Autodesk Fusion 360 part; units mm, degrees
(part 2 of 2)
sketch "Sketch2 (2)" plane through (0, 0, 0) normal (0, 0, 1) x (1, 0, 0) in component "Spur Gear (8 teeth)"
  spline S0 degree 5 poles (4.6675, -1.001) (4.6721, -1.0019) (4.6813, -1.0037) (4.6952, -1.0059) (4.7138, -1.0078) (4.7373, -1.0088) (4.7609, -1.0089) (4.7846, -1.0084) (4.8084, -1.0076) (4.8323, -1.0065) (4.8562, -1.0051) (4.8801, -1.0035) (4.9041, -1.0014) (4.9282, -0.9988) (4.9523, -0.9957) (4.9764, -0.9922) (5.0006, -0.9883) (5.0248, -0.9841) (5.049, -0.9795) (5.0733, -0.9747) (5.0975, -0.9696) (5.1218, -0.9642) (5.1461, -0.9584) (5.1705, -0.9524) (5.1948, -0.946) (5.2191, -0.9393) (5.2435, -0.9324) (5.2679, -0.9251) (5.2922, -0.9176) (5.3166, -0.9098) (5.3409, -0.9017) (5.3653, -0.8934) (5.3896, -0.8848) (5.414, -0.8759) (5.4383, -0.8668) (5.4626, -0.8574) (5.4869, -0.8477) (5.5112, -0.8378) (5.5355, -0.8277) (5.5598, -0.8173) (5.584, -0.8066) (5.6082, -0.7957) (5.6324, -0.7845) (5.6566, -0.7731) (5.6808, -0.7615) (5.7049, -0.7496) (5.729, -0.7375) (5.7531, -0.7252) (5.7771, -0.7126) (5.8011, -0.6997) (5.825, -0.6867) (5.849, -0.6734) (5.8729, -0.6599) (5.8967, -0.6462) (5.9205, -0.6322) (5.9443, -0.618) (5.968, -0.6036) (5.9917, -0.589) (6.0153, -0.5741) (6.0389, -0.559) (6.0625, -0.5438) (6.086, -0.5282) (6.1094, -0.5125) (6.1328, -0.4966) (6.1561, -0.4804) (6.1794, -0.464) (6.2026, -0.4475) (6.2258, -0.4307) (6.2489, -0.4137) (6.2719, -0.3965) (6.2949, -0.379) (6.3133, -0.3649) (6.327, -0.3543) (6.3361, -0.3471) (6.3407, -0.3435) knots 0 0 0 0 0 0 0.01428571 0.02857143 0.04285714 0.05714286 0.07142857 0.08571429 0.1 0.11428571 0.12857143 0.14285714 0.15714286 0.17142857 0.18571429 0.2 0.21428571 0.22857143 0.24285714 0.25714286 0.27142857 0.28571429 0.3 0.31428571 0.32857143 0.34285714 0.35714286 0.37142857 0.38571429 0.4 0.41428571 0.42857143 0.44285714 0.45714286 0.47142857 0.48571429 0.5 0.51428571 0.52857143 0.54285714 0.55714286 0.57142857 0.58571429 0.6 0.61428571 0.62857143 0.64285714 0.65714286 0.67142857 0.68571429 0.7 0.71428571 0.72857143 0.74285714 0.75714286 0.77142857 0.78571429 0.8 0.81428571 0.82857143 0.84285714 0.85714286 0.87142857 0.88571429 0.9 0.91428571 0.92857143 0.94285714 0.95714286 0.97142857 0.98571429 1 1 1 1 1 1
  spline S1 degree 5 poles (4.6675, 1.001) (4.6721, 1.0019) (4.6813, 1.0037) (4.6952, 1.0059) (4.7138, 1.0078) (4.7373, 1.0088) (4.7609, 1.0089) (4.7846, 1.0084) (4.8084, 1.0076) (4.8323, 1.0065) (4.8562, 1.0051) (4.8801, 1.0035) (4.9041, 1.0014) (4.9282, 0.9988) (4.9523, 0.9957) (4.9764, 0.9922) (5.0006, 0.9883) (5.0248, 0.9841) (5.049, 0.9795) (5.0733, 0.9747) (5.0975, 0.9696) (5.1218, 0.9642) (5.1461, 0.9584) (5.1705, 0.9524) (5.1948, 0.946) (5.2191, 0.9393) (5.2435, 0.9324) (5.2679, 0.9251) (5.2922, 0.9176) (5.3166, 0.9098) (5.3409, 0.9017) (5.3653, 0.8934) (5.3896, 0.8848) (5.414, 0.8759) (5.4383, 0.8668) (5.4626, 0.8574) (5.4869, 0.8477) (5.5112, 0.8378) (5.5355, 0.8277) (5.5598, 0.8173) (5.584, 0.8066) (5.6082, 0.7957) (5.6324, 0.7845) (5.6566, 0.7731) (5.6808, 0.7615) (5.7049, 0.7496) (5.729, 0.7375) (5.7531, 0.7252) (5.7771, 0.7126) (5.8011, 0.6997) (5.825, 0.6867) (5.849, 0.6734) (5.8729, 0.6599) (5.8967, 0.6462) (5.9205, 0.6322) (5.9443, 0.618) (5.968, 0.6036) (5.9917, 0.589) (6.0153, 0.5741) (6.0389, 0.559) (6.0625, 0.5438) (6.086, 0.5282) (6.1094, 0.5125) (6.1328, 0.4966) (6.1561, 0.4804) (6.1794, 0.464) (6.2026, 0.4475) (6.2258, 0.4307) (6.2489, 0.4137) (6.2719, 0.3965) (6.2949, 0.379) (6.3133, 0.3649) (6.327, 0.3543) (6.3361, 0.3471) (6.3407, 0.3435) knots 0 0 0 0 0 0 0.01428571 0.02857143 0.04285714 0.05714286 0.07142857 0.08571429 0.1 0.11428571 0.12857143 0.14285714 0.15714286 0.17142857 0.18571429 0.2 0.21428571 0.22857143 0.24285714 0.25714286 0.27142857 0.28571429 0.3 0.31428571 0.32857143 0.34285714 0.35714286 0.37142857 0.38571429 0.4 0.41428571 0.42857143 0.44285714 0.45714286 0.47142857 0.48571429 0.5 0.51428571 0.52857143 0.54285714 0.55714286 0.57142857 0.58571429 0.6 0.61428571 0.62857143 0.64285714 0.65714286 0.67142857 0.68571429 0.7 0.71428571 0.72857143 0.74285714 0.75714286 0.77142857 0.78571429 0.8 0.81428571 0.82857143 0.84285714 0.85714286 0.87142857 0.88571429 0.9 0.91428571 0.92857143 0.94285714 0.95714286 0.97142857 0.98571429 1 1 1 1 1 1
  arc A0 (6.3407, -0.3435) -> (6.3407, 0.3435) centre (0, 0) ccw
  line L0 (3.4175, -0.735) -> (4.6675, -1.001)
  line L1 (3.4175, 0.735) -> (4.6675, 1.001)
  line L2 (3.4175, -0.735) -> (3.4175, 0.735)
  point P0 (4.781, -1.0084)
  point P1 (4.8974, -1.0019)
  point P2 (5.0155, -0.9856)
  point P3 (5.1349, -0.961)
  point P4 (5.2552, -0.9289)
  point P5 (5.3761, -0.8895)
  point P6 (5.4975, -0.8434)
  point P7 (5.6191, -0.7907)
  point P8 (5.7406, -0.7315)
  point P9 (5.8619, -0.6661)
  point P10 (5.9827, -0.5945)
  point P11 (6.103, -0.5168)
  point P12 (6.2223, -0.4331)
  point P13 (4.781, 1.0084)
  point P14 (4.8974, 1.0019)
  point P15 (5.0155, 0.9856)
  point P16 (5.1349, 0.961)
  point P17 (5.2552, 0.9289)
  point P18 (5.3761, 0.8895)
  point P19 (5.4975, 0.8434)
  point P20 (5.6191, 0.7907)
  point P21 (5.7406, 0.7315)
  point P22 (5.8619, 0.6661)
  point P23 (5.9827, 0.5945)
  point P24 (6.103, 0.5168)
  point P25 (6.2223, 0.4331)
extrude "Extrude2" add sketch "Sketch2 (2)" along normal blind 7.62 in component "Spur Gear (8 teeth)"
fillet "Fillet1" radius 0.254 2 edges at (3.4268, -0.737, 3.81) (3.4268, 0.737, 3.81) in component "Spur Gear (8 teeth)"
pattern_circular "C-Pattern1" count 8 over 360 about axis through (0, 0, 0) along (0, 0, 1) of "Extrude2", "Fillet1" in component "Spur Gear (8 teeth)"
sketch "Sketch3" plane through (0, 0, 0) normal (0, 0, 1) x (1, 0, 0) in component "Spur Gear (8 teeth)"
  circle A0 centre (0, 0) radius 5.08 construction
sketch "Sketch3 (2)" plane through (0, 0, 0) normal (0, 0, -1) x (-1, 0, 0)
  circle A0 centre (0, 0) radius 3.175
  arc A1 (-0.7879, -3.6664) -> (-0.9664, -3.3694) centre (-1.0364, -3.6135) ccw
  line L0 (-0.7879, -3.6664) -> (-1.001, -4.6675)
  spline S0 degree 5 poles (-1.001, -4.6675) (-1.0019, -4.6721) (-1.0037, -4.6813) (-1.0059, -4.6952) (-1.0078, -4.7138) (-1.0088, -4.7373) (-1.0089, -4.7609) (-1.0084, -4.7846) (-1.0076, -4.8084) (-1.0065, -4.8323) (-1.0051, -4.8562) (-1.0035, -4.8801) (-1.0014, -4.9041) (-0.9988, -4.9282) (-0.9957, -4.9523) (-0.9922, -4.9764) (-0.9883, -5.0006) (-0.9841, -5.0248) (-0.9795, -5.049) (-0.9747, -5.0733) (-0.9696, -5.0975) (-0.9642, -5.1218) (-0.9584, -5.1461) (-0.9524, -5.1705) (-0.946, -5.1948) (-0.9393, -5.2191) (-0.9324, -5.2435) (-0.9251, -5.2679) (-0.9176, -5.2922) (-0.9098, -5.3166) (-0.9017, -5.3409) (-0.8934, -5.3653) (-0.8848, -5.3896) (-0.8759, -5.414) (-0.8668, -5.4383) (-0.8574, -5.4626) (-0.8477, -5.4869) (-0.8378, -5.5112) (-0.8277, -5.5355) (-0.8173, -5.5598) (-0.8066, -5.584) (-0.7957, -5.6082) (-0.7845, -5.6324) (-0.7731, -5.6566) (-0.7615, -5.6808) (-0.7496, -5.7049) (-0.7375, -5.729) (-0.7252, -5.7531) (-0.7126, -5.7771) (-0.6997, -5.8011) (-0.6867, -5.825) (-0.6734, -5.849) (-0.6599, -5.8729) (-0.6462, -5.8967) (-0.6322, -5.9205) (-0.618, -5.9443) (-0.6036, -5.968) (-0.589, -5.9917) (-0.5741, -6.0153) (-0.559, -6.0389) (-0.5438, -6.0625) (-0.5282, -6.086) (-0.5125, -6.1094) (-0.4966, -6.1328) (-0.4804, -6.1561) (-0.464, -6.1794) (-0.4475, -6.2026) (-0.4307, -6.2258) (-0.4137, -6.2489) (-0.3965, -6.2719) (-0.379, -6.2949) (-0.3649, -6.3133) (-0.3543, -6.327) (-0.3471, -6.3361) (-0.3435, -6.3407) knots 0 0 0 0 0 0 0.01428571 0.02857143 0.04285714 0.05714286 0.07142857 0.08571429 0.1 0.11428571 0.12857143 0.14285714 0.15714286 0.17142857 0.18571429 0.2 0.21428571 0.22857143 0.24285714 0.25714286 0.27142857 0.28571429 0.3 0.31428571 0.32857143 0.34285714 0.35714286 0.37142857 0.38571429 0.4 0.41428571 0.42857143 0.44285714 0.45714286 0.47142857 0.48571429 0.5 0.51428571 0.52857143 0.54285714 0.55714286 0.57142857 0.58571429 0.6 0.61428571 0.62857143 0.64285714 0.65714286 0.67142857 0.68571429 0.7 0.71428571 0.72857143 0.74285714 0.75714286 0.77142857 0.78571429 0.8 0.81428571 0.82857143 0.84285714 0.85714286 0.87142857 0.88571429 0.9 0.91428571 0.92857143 0.94285714 0.95714286 0.97142857 0.98571429 1 1 1 1 1 1
  arc A2 (-0.3435, -6.3407) -> (0.3435, -6.3407) centre (0, 0) ccw
  spline S1 degree 5 poles (1.001, -4.6675) (1.0019, -4.6721) (1.0037, -4.6813) (1.0059, -4.6952) (1.0078, -4.7138) (1.0088, -4.7373) (1.0089, -4.7609) (1.0084, -4.7846) (1.0076, -4.8084) (1.0065, -4.8323) (1.0051, -4.8562) (1.0035, -4.8801) (1.0014, -4.9041) (0.9988, -4.9282) (0.9957, -4.9523) (0.9922, -4.9764) (0.9883, -5.0006) (0.9841, -5.0248) (0.9795, -5.049) (0.9747, -5.0733) (0.9696, -5.0975) (0.9642, -5.1218) (0.9584, -5.1461) (0.9524, -5.1705) (0.946, -5.1948) (0.9393, -5.2191) (0.9324, -5.2435) (0.9251, -5.2679) (0.9176, -5.2922) (0.9098, -5.3166) (0.9017, -5.3409) (0.8934, -5.3653) (0.8848, -5.3896) (0.8759, -5.414) (0.8668, -5.4383) (0.8574, -5.4626) (0.8477, -5.4869) (0.8378, -5.5112) (0.8277, -5.5355) (0.8173, -5.5598) (0.8066, -5.584) (0.7957, -5.6082) (0.7845, -5.6324) (0.7731, -5.6566) (0.7615, -5.6808) (0.7496, -5.7049) (0.7375, -5.729) (0.7252, -5.7531) (0.7126, -5.7771) (0.6997, -5.8011) (0.6867, -5.825) (0.6734, -5.849) (0.6599, -5.8729) (0.6462, -5.8967) (0.6322, -5.9205) (0.618, -5.9443) (0.6036, -5.968) (0.589, -5.9917) (0.5741, -6.0153) (0.559, -6.0389) (0.5438, -6.0625) (0.5282, -6.086) (0.5125, -6.1094) (0.4966, -6.1328) (0.4804, -6.1561) (0.464, -6.1794) (0.4475, -6.2026) (0.4307, -6.2258) (0.4137, -6.2489) (0.3965, -6.2719) (0.379, -6.2949) (0.3649, -6.3133) (0.3543, -6.327) (0.3471, -6.3361) (0.3435, -6.3407) knots 0 0 0 0 0 0 0.01428571 0.02857143 0.04285714 0.05714286 0.07142857 0.08571429 0.1 0.11428571 0.12857143 0.14285714 0.15714286 0.17142857 0.18571429 0.2 0.21428571 0.22857143 0.24285714 0.25714286 0.27142857 0.28571429 0.3 0.31428571 0.32857143 0.34285714 0.35714286 0.37142857 0.38571429 0.4 0.41428571 0.42857143 0.44285714 0.45714286 0.47142857 0.48571429 0.5 0.51428571 0.52857143 0.54285714 0.55714286 0.57142857 0.58571429 0.6 0.61428571 0.62857143 0.64285714 0.65714286 0.67142857 0.68571429 0.7 0.71428571 0.72857143 0.74285714 0.75714286 0.77142857 0.78571429 0.8 0.81428571 0.82857143 0.84285714 0.85714286 0.87142857 0.88571429 0.9 0.91428571 0.92857143 0.94285714 0.95714286 0.97142857 0.98571429 1 1 1 1 1 1
  line L1 (1.001, -4.6675) -> (0.7879, -3.6664)
  arc A3 (0.9664, -3.3694) -> (0.7879, -3.6664) centre (1.0364, -3.6135) ccw
  arc A4 (0.9664, -3.3694) -> (1.6992, -3.0658) centre (0, 0) ccw
  arc A5 (2.0354, -3.1497) -> (1.6992, -3.0658) centre (1.8223, -3.288) ccw
  line L2 (2.0354, -3.1497) -> (2.5926, -4.0082)
  spline S2 degree 5 poles (2.5926, -4.0082) (2.5952, -4.0122) (2.6004, -4.0199) (2.6087, -4.0313) (2.6205, -4.0458) (2.6364, -4.0631) (2.6531, -4.0799) (2.6702, -4.0963) (2.6876, -4.1125) (2.7053, -4.1286) (2.7231, -4.1446) (2.7412, -4.1603) (2.7596, -4.1758) (2.7785, -4.191) (2.7977, -4.2059) (2.8172, -4.2204) (2.8371, -4.2348) (2.8572, -4.2489) (2.8776, -4.2628) (2.8981, -4.2766) (2.9189, -4.2901) (2.9399, -4.3035) (2.9612, -4.3166) (2.9826, -4.3295) (3.0043, -4.3422) (3.0263, -4.3547) (3.0484, -4.367) (3.0708, -4.3791) (3.0933, -4.391) (3.1161, -4.4027) (3.139, -4.4142) (3.1621, -4.4256) (3.1854, -4.4367) (3.2089, -4.4476) (3.2326, -4.4584) (3.2564, -4.4689) (3.2804, -4.4793) (3.3046, -4.4895) (3.329, -4.4994) (3.3535, -4.5092) (3.3782, -4.5188) (3.403, -4.5283) (3.428, -4.5375) (3.4531, -4.5465) (3.4784, -4.5554) (3.5039, -4.564) (3.5295, -4.5725) (3.5553, -4.5808) (3.5812, -4.5889) (3.6072, -4.5968) (3.6334, -4.6045) (3.6597, -4.612) (3.6861, -4.6194) (3.7127, -4.6265) (3.7394, -4.6335) (3.7662, -4.6403) (3.7932, -4.6468) (3.8203, -4.6532) (3.8475, -4.6595) (3.8749, -4.6655) (3.9023, -4.6713) (3.9299, -4.677) (3.9576, -4.6824) (3.9854, -4.6877) (4.0133, -4.6927) (4.0414, -4.6976) (4.0695, -4.7023) (4.0978, -4.7068) (4.1261, -4.7112) (4.1546, -4.7153) (4.1832, -4.7192) (4.2061, -4.7222) (4.2234, -4.7244) (4.2349, -4.7258) (4.2406, -4.7265) knots 0 0 0 0 0 0 0.01428571 0.02857143 0.04285714 0.05714286 0.07142857 0.08571429 0.1 0.11428571 0.12857143 0.14285714 0.15714286 0.17142857 0.18571429 0.2 0.21428571 0.22857143 0.24285714 0.25714286 0.27142857 0.28571429 0.3 0.31428571 0.32857143 0.34285714 0.35714286 0.37142857 0.38571429 0.4 0.41428571 0.42857143 0.44285714 0.45714286 0.47142857 0.48571429 0.5 0.51428571 0.52857143 0.54285714 0.55714286 0.57142857 0.58571429 0.6 0.61428571 0.62857143 0.64285714 0.65714286 0.67142857 0.68571429 0.7 0.71428571 0.72857143 0.74285714 0.75714286 0.77142857 0.78571429 0.8 0.81428571 0.82857143 0.84285714 0.85714286 0.87142857 0.88571429 0.9 0.91428571 0.92857143 0.94285714 0.95714286 0.97142857 0.98571429 1 1 1 1 1 1
  arc A6 (4.2406, -4.7265) -> (4.7265, -4.2406) centre (0, 0) ccw
  spline S3 degree 5 poles (4.0082, -2.5926) (4.0122, -2.5952) (4.0199, -2.6004) (4.0313, -2.6087) (4.0458, -2.6205) (4.0631, -2.6364) (4.0799, -2.6531) (4.0963, -2.6702) (4.1125, -2.6876) (4.1286, -2.7053) (4.1446, -2.7231) (4.1603, -2.7412) (4.1758, -2.7596) (4.191, -2.7785) (4.2059, -2.7977) (4.2204, -2.8172) (4.2348, -2.8371) (4.2489, -2.8572) (4.2628, -2.8776) (4.2766, -2.8981) (4.2901, -2.9189) (4.3035, -2.9399) (4.3166, -2.9612) (4.3295, -2.9826) (4.3422, -3.0043) (4.3547, -3.0263) (4.367, -3.0484) (4.3791, -3.0708) (4.391, -3.0933) (4.4027, -3.1161) (4.4142, -3.139) (4.4256, -3.1621) (4.4367, -3.1854) (4.4476, -3.2089) (4.4584, -3.2326) (4.4689, -3.2564) (4.4793, -3.2804) (4.4895, -3.3046) (4.4994, -3.329) (4.5092, -3.3535) (4.5188, -3.3782) (4.5283, -3.403) (4.5375, -3.428) (4.5465, -3.4531) (4.5554, -3.4784) (4.564, -3.5039) (4.5725, -3.5295) (4.5808, -3.5553) (4.5889, -3.5812) (4.5968, -3.6072) (4.6045, -3.6334) (4.612, -3.6597) (4.6194, -3.6861) (4.6265, -3.7127) (4.6335, -3.7394) (4.6403, -3.7662) (4.6468, -3.7932) (4.6532, -3.8203) (4.6595, -3.8475) (4.6655, -3.8749) (4.6713, -3.9023) (4.677, -3.9299) (4.6824, -3.9576) (4.6877, -3.9854) (4.6927, -4.0133) (4.6976, -4.0414) (4.7023, -4.0695) (4.7068, -4.0978) (4.7112, -4.1261) (4.7153, -4.1546) (4.7192, -4.1832) (4.7222, -4.2061) (4.7244, -4.2234) (4.7258, -4.2349) (4.7265, -4.2406) knots 0 0 0 0 0 0 0.01428571 0.02857143 0.04285714 0.05714286 0.07142857 0.08571429 0.1 0.11428571 0.12857143 0.14285714 0.15714286 0.17142857 0.18571429 0.2 0.21428571 0.22857143 0.24285714 0.25714286 0.27142857 0.28571429 0.3 0.31428571 0.32857143 0.34285714 0.35714286 0.37142857 0.38571429 0.4 0.41428571 0.42857143 0.44285714 0.45714286 0.47142857 0.48571429 0.5 0.51428571 0.52857143 0.54285714 0.55714286 0.57142857 0.58571429 0.6 0.61428571 0.62857143 0.64285714 0.65714286 0.67142857 0.68571429 0.7 0.71428571 0.72857143 0.74285714 0.75714286 0.77142857 0.78571429 0.8 0.81428571 0.82857143 0.84285714 0.85714286 0.87142857 0.88571429 0.9 0.91428571 0.92857143 0.94285714 0.95714286 0.97142857 0.98571429 1 1 1 1 1 1
  line L3 (4.0082, -2.5926) -> (3.1497, -2.0354)
  arc A7 (3.0658, -1.6992) -> (3.1497, -2.0354) centre (3.288, -1.8223) ccw
  arc A8 (3.0658, -1.6992) -> (3.3694, -0.9664) centre (0, 0) ccw
  arc A9 (3.6664, -0.7879) -> (3.3694, -0.9664) centre (3.6135, -1.0364) ccw
  line L4 (3.6664, -0.7879) -> (4.6675, -1.001)
  spline S4 degree 5 poles (4.6675, -1.001) (4.6721, -1.0019) (4.6813, -1.0037) (4.6952, -1.0059) (4.7138, -1.0078) (4.7373, -1.0088) (4.7609, -1.0089) (4.7846, -1.0084) (4.8084, -1.0076) (4.8323, -1.0065) (4.8562, -1.0051) (4.8801, -1.0035) (4.9041, -1.0014) (4.9282, -0.9988) (4.9523, -0.9957) (4.9764, -0.9922) (5.0006, -0.9883) (5.0248, -0.9841) (5.049, -0.9795) (5.0733, -0.9747) (5.0975, -0.9696) (5.1218, -0.9642) (5.1461, -0.9584) (5.1705, -0.9524) (5.1948, -0.946) (5.2191, -0.9393) (5.2435, -0.9324) (5.2679, -0.9251) (5.2922, -0.9176) (5.3166, -0.9098) (5.3409, -0.9017) (5.3653, -0.8934) (5.3896, -0.8848) (5.414, -0.8759) (5.4383, -0.8668) (5.4626, -0.8574) (5.4869, -0.8477) (5.5112, -0.8378) (5.5355, -0.8277) (5.5598, -0.8173) (5.584, -0.8066) (5.6082, -0.7957) (5.6324, -0.7845) (5.6566, -0.7731) (5.6808, -0.7615) (5.7049, -0.7496) (5.729, -0.7375) (5.7531, -0.7252) (5.7771, -0.7126) (5.8011, -0.6997) (5.825, -0.6867) (5.849, -0.6734) (5.8729, -0.6599) (5.8967, -0.6462) (5.9205, -0.6322) (5.9443, -0.618) (5.968, -0.6036) (5.9917, -0.589) (6.0153, -0.5741) (6.0389, -0.559) (6.0625, -0.5438) (6.086, -0.5282) (6.1094, -0.5125) (6.1328, -0.4966) (6.1561, -0.4804) (6.1794, -0.464) (6.2026, -0.4475) (6.2258, -0.4307) (6.2489, -0.4137) (6.2719, -0.3965) (6.2949, -0.379) (6.3133, -0.3649) (6.327, -0.3543) (6.3361, -0.3471) (6.3407, -0.3435) knots 0 0 0 0 0 0 0.01428571 0.02857143 0.04285714 0.05714286 0.07142857 0.08571429 0.1 0.11428571 0.12857143 0.14285714 0.15714286 0.17142857 0.18571429 0.2 0.21428571 0.22857143 0.24285714 0.25714286 0.27142857 0.28571429 0.3 0.31428571 0.32857143 0.34285714 0.35714286 0.37142857 0.38571429 0.4 0.41428571 0.42857143 0.44285714 0.45714286 0.47142857 0.48571429 0.5 0.51428571 0.52857143 0.54285714 0.55714286 0.57142857 0.58571429 0.6 0.61428571 0.62857143 0.64285714 0.65714286 0.67142857 0.68571429 0.7 0.71428571 0.72857143 0.74285714 0.75714286 0.77142857 0.78571429 0.8 0.81428571 0.82857143 0.84285714 0.85714286 0.87142857 0.88571429 0.9 0.91428571 0.92857143 0.94285714 0.95714286 0.97142857 0.98571429 1 1 1 1 1 1
  arc A10 (6.3407, -0.3435) -> (6.3407, 0.3435) centre (0, 0) ccw
  spline S5 degree 5 poles (4.6675, 1.001) (4.6721, 1.0019) (4.6813, 1.0037) (4.6952, 1.0059) (4.7138, 1.0078) (4.7373, 1.0088) (4.7609, 1.0089) (4.7846, 1.0084) (4.8084, 1.0076) (4.8323, 1.0065) (4.8562, 1.0051) (4.8801, 1.0035) (4.9041, 1.0014) (4.9282, 0.9988) (4.9523, 0.9957) (4.9764, 0.9922) (5.0006, 0.9883) (5.0248, 0.9841) (5.049, 0.9795) (5.0733, 0.9747) (5.0975, 0.9696) (5.1218, 0.9642) (5.1461, 0.9584) (5.1705, 0.9524) (5.1948, 0.946) (5.2191, 0.9393) (5.2435, 0.9324) (5.2679, 0.9251) (5.2922, 0.9176) (5.3166, 0.9098) (5.3409, 0.9017) (5.3653, 0.8934) (5.3896, 0.8848) (5.414, 0.8759) (5.4383, 0.8668) (5.4626, 0.8574) (5.4869, 0.8477) (5.5112, 0.8378) (5.5355, 0.8277) (5.5598, 0.8173) (5.584, 0.8066) (5.6082, 0.7957) (5.6324, 0.7845) (5.6566, 0.7731) (5.6808, 0.7615) (5.7049, 0.7496) (5.729, 0.7375) (5.7531, 0.7252) (5.7771, 0.7126) (5.8011, 0.6997) (5.825, 0.6867) (5.849, 0.6734) (5.8729, 0.6599) (5.8967, 0.6462) (5.9205, 0.6322) (5.9443, 0.618) (5.968, 0.6036) (5.9917, 0.589) (6.0153, 0.5741) (6.0389, 0.559) (6.0625, 0.5438) (6.086, 0.5282) (6.1094, 0.5125) (6.1328, 0.4966) (6.1561, 0.4804) (6.1794, 0.464) (6.2026, 0.4475) (6.2258, 0.4307) (6.2489, 0.4137) (6.2719, 0.3965) (6.2949, 0.379) (6.3133, 0.3649) (6.327, 0.3543) (6.3361, 0.3471) (6.3407, 0.3435) knots 0 0 0 0 0 0 0.01428571 0.02857143 0.04285714 0.05714286 0.07142857 0.08571429 0.1 0.11428571 0.12857143 0.14285714 0.15714286 0.17142857 0.18571429 0.2 0.21428571 0.22857143 0.24285714 0.25714286 0.27142857 0.28571429 0.3 0.31428571 0.32857143 0.34285714 0.35714286 0.37142857 0.38571429 0.4 0.41428571 0.42857143 0.44285714 0.45714286 0.47142857 0.48571429 0.5 0.51428571 0.52857143 0.54285714 0.55714286 0.57142857 0.58571429 0.6 0.61428571 0.62857143 0.64285714 0.65714286 0.67142857 0.68571429 0.7 0.71428571 0.72857143 0.74285714 0.75714286 0.77142857 0.78571429 0.8 0.81428571 0.82857143 0.84285714 0.85714286 0.87142857 0.88571429 0.9 0.91428571 0.92857143 0.94285714 0.95714286 0.97142857 0.98571429 1 1 1 1 1 1
  line L5 (4.6675, 1.001) -> (3.6664, 0.7879)
  arc A11 (3.3694, 0.9664) -> (3.6664, 0.7879) centre (3.6135, 1.0364) ccw
  arc A12 (3.3694, 0.9664) -> (3.0658, 1.6992) centre (0, 0) ccw
  arc A13 (3.1497, 2.0354) -> (3.0658, 1.6992) centre (3.288, 1.8223) ccw
  line L6 (3.1497, 2.0354) -> (4.0082, 2.5926)
  spline S6 degree 5 poles (4.0082, 2.5926) (4.0122, 2.5952) (4.0199, 2.6004) (4.0313, 2.6087) (4.0458, 2.6205) (4.0631, 2.6364) (4.0799, 2.6531) (4.0963, 2.6702) (4.1125, 2.6876) (4.1286, 2.7053) (4.1446, 2.7231) (4.1603, 2.7412) (4.1758, 2.7596) (4.191, 2.7785) (4.2059, 2.7977) (4.2204, 2.8172) (4.2348, 2.8371) (4.2489, 2.8572) (4.2628, 2.8776) (4.2766, 2.8981) (4.2901, 2.9189) (4.3035, 2.9399) (4.3166, 2.9612) (4.3295, 2.9826) (4.3422, 3.0043) (4.3547, 3.0263) (4.367, 3.0484) (4.3791, 3.0708) (4.391, 3.0933) (4.4027, 3.1161) (4.4142, 3.139) (4.4256, 3.1621) (4.4367, 3.1854) (4.4476, 3.2089) (4.4584, 3.2326) (4.4689, 3.2564) (4.4793, 3.2804) (4.4895, 3.3046) (4.4994, 3.329) (4.5092, 3.3535) (4.5188, 3.3782) (4.5283, 3.403) (4.5375, 3.428) (4.5465, 3.4531) (4.5554, 3.4784) (4.564, 3.5039) (4.5725, 3.5295) (4.5808, 3.5553) (4.5889, 3.5812) (4.5968, 3.6072) (4.6045, 3.6334) (4.612, 3.6597) (4.6194, 3.6861) (4.6265, 3.7127) (4.6335, 3.7394) (4.6403, 3.7662) (4.6468, 3.7932) (4.6532, 3.8203) (4.6595, 3.8475) (4.6655, 3.8749) (4.6713, 3.9023) (4.677, 3.9299) (4.6824, 3.9576) (4.6877, 3.9854) (4.6927, 4.0133) (4.6976, 4.0414) (4.7023, 4.0695) (4.7068, 4.0978) (4.7112, 4.1261) (4.7153, 4.1546) (4.7192, 4.1832) (4.7222, 4.2061) (4.7244, 4.2234) (4.7258, 4.2349) (4.7265, 4.2406) knots 0 0 0 0 0 0 0.01428571 0.02857143 0.04285714 0.05714286 0.07142857 0.08571429 0.1 0.11428571 0.12857143 0.14285714 0.15714286 0.17142857 0.18571429 0.2 0.21428571 0.22857143 0.24285714 0.25714286 0.27142857 0.28571429 0.3 0.31428571 0.32857143 0.34285714 0.35714286 0.37142857 0.38571429 0.4 0.41428571 0.42857143 0.44285714 0.45714286 0.47142857 0.48571429 0.5 0.51428571 0.52857143 0.54285714 0.55714286 0.57142857 0.58571429 0.6 0.61428571 0.62857143 0.64285714 0.65714286 0.67142857 0.68571429 0.7 0.71428571 0.72857143 0.74285714 0.75714286 0.77142857 0.78571429 0.8 0.81428571 0.82857143 0.84285714 0.85714286 0.87142857 0.88571429 0.9 0.91428571 0.92857143 0.94285714 0.95714286 0.97142857 0.98571429 1 1 1 1 1 1
  arc A14 (4.7265, 4.2406) -> (4.2406, 4.7265) centre (0, 0) ccw
  spline S7 degree 5 poles (2.5926, 4.0082) (2.5952, 4.0122) (2.6004, 4.0199) (2.6087, 4.0313) (2.6205, 4.0458) (2.6364, 4.0631) (2.6531, 4.0799) (2.6702, 4.0963) (2.6876, 4.1125) (2.7053, 4.1286) (2.7231, 4.1446) (2.7412, 4.1603) (2.7596, 4.1758) (2.7785, 4.191) (2.7977, 4.2059) (2.8172, 4.2204) (2.8371, 4.2348) (2.8572, 4.2489) (2.8776, 4.2628) (2.8981, 4.2766) (2.9189, 4.2901) (2.9399, 4.3035) (2.9612, 4.3166) (2.9826, 4.3295) (3.0043, 4.3422) (3.0263, 4.3547) (3.0484, 4.367) (3.0708, 4.3791) (3.0933, 4.391) (3.1161, 4.4027) (3.139, 4.4142) (3.1621, 4.4256) (3.1854, 4.4367) (3.2089, 4.4476) (3.2326, 4.4584) (3.2564, 4.4689) (3.2804, 4.4793) (3.3046, 4.4895) (3.329, 4.4994) (3.3535, 4.5092) (3.3782, 4.5188) (3.403, 4.5283) (3.428, 4.5375) (3.4531, 4.5465) (3.4784, 4.5554) (3.5039, 4.564) (3.5295, 4.5725) (3.5553, 4.5808) (3.5812, 4.5889) (3.6072, 4.5968) (3.6334, 4.6045) (3.6597, 4.612) (3.6861, 4.6194) (3.7127, 4.6265) (3.7394, 4.6335) (3.7662, 4.6403) (3.7932, 4.6468) (3.8203, 4.6532) (3.8475, 4.6595) (3.8749, 4.6655) (3.9023, 4.6713) (3.9299, 4.677) (3.9576, 4.6824) (3.9854, 4.6877) (4.0133, 4.6927) (4.0414, 4.6976) (4.0695, 4.7023) (4.0978, 4.7068) (4.1261, 4.7112) (4.1546, 4.7153) (4.1832, 4.7192) (4.2061, 4.7222) (4.2234, 4.7244) (4.2349, 4.7258) (4.2406, 4.7265) knots 0 0 0 0 0 0 0.01428571 0.02857143 0.04285714 0.05714286 0.07142857 0.08571429 0.1 0.11428571 0.12857143 0.14285714 0.15714286 0.17142857 0.18571429 0.2 0.21428571 0.22857143 0.24285714 0.25714286 0.27142857 0.28571429 0.3 0.31428571 0.32857143 0.34285714 0.35714286 0.37142857 0.38571429 0.4 0.41428571 0.42857143 0.44285714 0.45714286 0.47142857 0.48571429 0.5 0.51428571 0.52857143 0.54285714 0.55714286 0.57142857 0.58571429 0.6 0.61428571 0.62857143 0.64285714 0.65714286 0.67142857 0.68571429 0.7 0.71428571 0.72857143 0.74285714 0.75714286 0.77142857 0.78571429 0.8 0.81428571 0.82857143 0.84285714 0.85714286 0.87142857 0.88571429 0.9 0.91428571 0.92857143 0.94285714 0.95714286 0.97142857 0.98571429 1 1 1 1 1 1
  line L7 (2.5926, 4.0082) -> (2.0354, 3.1497)
  arc A15 (1.6992, 3.0658) -> (2.0354, 3.1497) centre (1.8223, 3.288) ccw
  arc A16 (1.6992, 3.0658) -> (0.9664, 3.3694) centre (0, 0) ccw
  arc A17 (0.7879, 3.6664) -> (0.9664, 3.3694) centre (1.0364, 3.6135) ccw
  line L8 (0.7879, 3.6664) -> (1.001, 4.6675)
  spline S8 degree 5 poles (1.001, 4.6675) (1.0019, 4.6721) (1.0037, 4.6813) (1.0059, 4.6952) (1.0078, 4.7138) (1.0088, 4.7373) (1.0089, 4.7609) (1.0084, 4.7846) (1.0076, 4.8084) (1.0065, 4.8323) (1.0051, 4.8562) (1.0035, 4.8801) (1.0014, 4.9041) (0.9988, 4.9282) (0.9957, 4.9523) (0.9922, 4.9764) (0.9883, 5.0006) (0.9841, 5.0248) (0.9795, 5.049) (0.9747, 5.0733) (0.9696, 5.0975) (0.9642, 5.1218) (0.9584, 5.1461) (0.9524, 5.1705) (0.946, 5.1948) (0.9393, 5.2191) (0.9324, 5.2435) (0.9251, 5.2679) (0.9176, 5.2922) (0.9098, 5.3166) (0.9017, 5.3409) (0.8934, 5.3653) (0.8848, 5.3896) (0.8759, 5.414) (0.8668, 5.4383) (0.8574, 5.4626) (0.8477, 5.4869) (0.8378, 5.5112) (0.8277, 5.5355) (0.8173, 5.5598) (0.8066, 5.584) (0.7957, 5.6082) (0.7845, 5.6324) (0.7731, 5.6566) (0.7615, 5.6808) (0.7496, 5.7049) (0.7375, 5.729) (0.7252, 5.7531) (0.7126, 5.7771) (0.6997, 5.8011) (0.6867, 5.825) (0.6734, 5.849) (0.6599, 5.8729) (0.6462, 5.8967) (0.6322, 5.9205) (0.618, 5.9443) (0.6036, 5.968) (0.589, 5.9917) (0.5741, 6.0153) (0.559, 6.0389) (0.5438, 6.0625) (0.5282, 6.086) (0.5125, 6.1094) (0.4966, 6.1328) (0.4804, 6.1561) (0.464, 6.1794) (0.4475, 6.2026) (0.4307, 6.2258) (0.4137, 6.2489) (0.3965, 6.2719) (0.379, 6.2949) (0.3649, 6.3133) (0.3543, 6.327) (0.3471, 6.3361) (0.3435, 6.3407) knots 0 0 0 0 0 0 0.01428571 0.02857143 0.04285714 0.05714286 0.07142857 0.08571429 0.1 0.11428571 0.12857143 0.14285714 0.15714286 0.17142857 0.18571429 0.2 0.21428571 0.22857143 0.24285714 0.25714286 0.27142857 0.28571429 0.3 0.31428571 0.32857143 0.34285714 0.35714286 0.37142857 0.38571429 0.4 0.41428571 0.42857143 0.44285714 0.45714286 0.47142857 0.48571429 0.5 0.51428571 0.52857143 0.54285714 0.55714286 0.57142857 0.58571429 0.6 0.61428571 0.62857143 0.64285714 0.65714286 0.67142857 0.68571429 0.7 0.71428571 0.72857143 0.74285714 0.75714286 0.77142857 0.78571429 0.8 0.81428571 0.82857143 0.84285714 0.85714286 0.87142857 0.88571429 0.9 0.91428571 0.92857143 0.94285714 0.95714286 0.97142857 0.98571429 1 1 1 1 1 1
  arc A18 (0.3435, 6.3407) -> (-0.3435, 6.3407) centre (0, 0) ccw
  spline S9 degree 5 poles (-1.001, 4.6675) (-1.0019, 4.6721) (-1.0037, 4.6813) (-1.0059, 4.6952) (-1.0078, 4.7138) (-1.0088, 4.7373) (-1.0089, 4.7609) (-1.0084, 4.7846) (-1.0076, 4.8084) (-1.0065, 4.8323) (-1.0051, 4.8562) (-1.0035, 4.8801) (-1.0014, 4.9041) (-0.9988, 4.9282) (-0.9957, 4.9523) (-0.9922, 4.9764) (-0.9883, 5.0006) (-0.9841, 5.0248) (-0.9795, 5.049) (-0.9747, 5.0733) (-0.9696, 5.0975) (-0.9642, 5.1218) (-0.9584, 5.1461) (-0.9524, 5.1705) (-0.946, 5.1948) (-0.9393, 5.2191) (-0.9324, 5.2435) (-0.9251, 5.2679) (-0.9176, 5.2922) (-0.9098, 5.3166) (-0.9017, 5.3409) (-0.8934, 5.3653) (-0.8848, 5.3896) (-0.8759, 5.414) (-0.8668, 5.4383) (-0.8574, 5.4626) (-0.8477, 5.4869) (-0.8378, 5.5112) (-0.8277, 5.5355) (-0.8173, 5.5598) (-0.8066, 5.584) (-0.7957, 5.6082) (-0.7845, 5.6324) (-0.7731, 5.6566) (-0.7615, 5.6808) (-0.7496, 5.7049) (-0.7375, 5.729) (-0.7252, 5.7531) (-0.7126, 5.7771) (-0.6997, 5.8011) (-0.6867, 5.825) (-0.6734, 5.849) (-0.6599, 5.8729) (-0.6462, 5.8967) (-0.6322, 5.9205) (-0.618, 5.9443) (-0.6036, 5.968) (-0.589, 5.9917) (-0.5741, 6.0153) (-0.559, 6.0389) (-0.5438, 6.0625) (-0.5282, 6.086) (-0.5125, 6.1094) (-0.4966, 6.1328) (-0.4804, 6.1561) (-0.464, 6.1794) (-0.4475, 6.2026) (-0.4307, 6.2258) (-0.4137, 6.2489) (-0.3965, 6.2719) (-0.379, 6.2949) (-0.3649, 6.3133) (-0.3543, 6.327) (-0.3471, 6.3361) (-0.3435, 6.3407) knots 0 0 0 0 0 0 0.01428571 0.02857143 0.04285714 0.05714286 0.07142857 0.08571429 0.1 0.11428571 0.12857143 0.14285714 0.15714286 0.17142857 0.18571429 0.2 0.21428571 0.22857143 0.24285714 0.25714286 0.27142857 0.28571429 0.3 0.31428571 0.32857143 0.34285714 0.35714286 0.37142857 0.38571429 0.4 0.41428571 0.42857143 0.44285714 0.45714286 0.47142857 0.48571429 0.5 0.51428571 0.52857143 0.54285714 0.55714286 0.57142857 0.58571429 0.6 0.61428571 0.62857143 0.64285714 0.65714286 0.67142857 0.68571429 0.7 0.71428571 0.72857143 0.74285714 0.75714286 0.77142857 0.78571429 0.8 0.81428571 0.82857143 0.84285714 0.85714286 0.87142857 0.88571429 0.9 0.91428571 0.92857143 0.94285714 0.95714286 0.97142857 0.98571429 1 1 1 1 1 1
  line L9 (-1.001, 4.6675) -> (-0.7879, 3.6664)
  arc A19 (-0.9664, 3.3694) -> (-0.7879, 3.6664) centre (-1.0364, 3.6135) ccw
  arc A20 (-0.9664, 3.3694) -> (-1.6992, 3.0658) centre (0, 0) ccw
  arc A21 (-2.0354, 3.1497) -> (-1.6992, 3.0658) centre (-1.8223, 3.288) ccw
  line L10 (-2.0354, 3.1497) -> (-2.5926, 4.0082)
  spline S10 degree 5 poles (-2.5926, 4.0082) (-2.5952, 4.0122) (-2.6004, 4.0199) (-2.6087, 4.0313) (-2.6205, 4.0458) (-2.6364, 4.0631) (-2.6531, 4.0799) (-2.6702, 4.0963) (-2.6876, 4.1125) (-2.7053, 4.1286) (-2.7231, 4.1446) (-2.7412, 4.1603) (-2.7596, 4.1758) (-2.7785, 4.191) (-2.7977, 4.2059) (-2.8172, 4.2204) (-2.8371, 4.2348) (-2.8572, 4.2489) (-2.8776, 4.2628) (-2.8981, 4.2766) (-2.9189, 4.2901) (-2.9399, 4.3035) (-2.9612, 4.3166) (-2.9826, 4.3295) (-3.0043, 4.3422) (-3.0263, 4.3547) (-3.0484, 4.367) (-3.0708, 4.3791) (-3.0933, 4.391) (-3.1161, 4.4027) (-3.139, 4.4142) (-3.1621, 4.4256) (-3.1854, 4.4367) (-3.2089, 4.4476) (-3.2326, 4.4584) (-3.2564, 4.4689) (-3.2804, 4.4793) (-3.3046, 4.4895) (-3.329, 4.4994) (-3.3535, 4.5092) (-3.3782, 4.5188) (-3.403, 4.5283) (-3.428, 4.5375) (-3.4531, 4.5465) (-3.4784, 4.5554) (-3.5039, 4.564) (-3.5295, 4.5725) (-3.5553, 4.5808) (-3.5812, 4.5889) (-3.6072, 4.5968) (-3.6334, 4.6045) (-3.6597, 4.612) (-3.6861, 4.6194) (-3.7127, 4.6265) (-3.7394, 4.6335) (-3.7662, 4.6403) (-3.7932, 4.6468) (-3.8203, 4.6532) (-3.8475, 4.6595) (-3.8749, 4.6655) (-3.9023, 4.6713) (-3.9299, 4.677) (-3.9576, 4.6824) (-3.9854, 4.6877) (-4.0133, 4.6927) (-4.0414, 4.6976) (-4.0695, 4.7023) (-4.0978, 4.7068) (-4.1261, 4.7112) (-4.1546, 4.7153) (-4.1832, 4.7192) (-4.2061, 4.7222) (-4.2234, 4.7244) (-4.2349, 4.7258) (-4.2406, 4.7265) knots 0 0 0 0 0 0 0.01428571 0.02857143 0.04285714 0.05714286 0.07142857 0.08571429 0.1 0.11428571 0.12857143 0.14285714 0.15714286 0.17142857 0.18571429 0.2 0.21428571 0.22857143 0.24285714 0.25714286 0.27142857 0.28571429 0.3 0.31428571 0.32857143 0.34285714 0.35714286 0.37142857 0.38571429 0.4 0.41428571 0.42857143 0.44285714 0.45714286 0.47142857 0.48571429 0.5 0.51428571 0.52857143 0.54285714 0.55714286 0.57142857 0.58571429 0.6 0.61428571 0.62857143 0.64285714 0.65714286 0.67142857 0.68571429 0.7 0.71428571 0.72857143 0.74285714 0.75714286 0.77142857 0.78571429 0.8 0.81428571 0.82857143 0.84285714 0.85714286 0.87142857 0.88571429 0.9 0.91428571 0.92857143 0.94285714 0.95714286 0.97142857 0.98571429 1 1 1 1 1 1
  arc A22 (-4.2406, 4.7265) -> (-4.7265, 4.2406) centre (0, 0) ccw
  spline S11 degree 5 poles (-4.0082, 2.5926) (-4.0122, 2.5952) (-4.0199, 2.6004) (-4.0313, 2.6087) (-4.0458, 2.6205) (-4.0631, 2.6364) (-4.0799, 2.6531) (-4.0963, 2.6702) (-4.1125, 2.6876) (-4.1286, 2.7053) (-4.1446, 2.7231) (-4.1603, 2.7412) (-4.1758, 2.7596) (-4.191, 2.7785) (-4.2059, 2.7977) (-4.2204, 2.8172) (-4.2348, 2.8371) (-4.2489, 2.8572) (-4.2628, 2.8776) (-4.2766, 2.8981) (-4.2901, 2.9189) (-4.3035, 2.9399) (-4.3166, 2.9612) (-4.3295, 2.9826) (-4.3422, 3.0043) (-4.3547, 3.0263) (-4.367, 3.0484) (-4.3791, 3.0708) (-4.391, 3.0933) (-4.4027, 3.1161) (-4.4142, 3.139) (-4.4256, 3.1621) (-4.4367, 3.1854) (-4.4476, 3.2089) (-4.4584, 3.2326) (-4.4689, 3.2564) (-4.4793, 3.2804) (-4.4895, 3.3046) (-4.4994, 3.329) (-4.5092, 3.3535) (-4.5188, 3.3782) (-4.5283, 3.403) (-4.5375, 3.428) (-4.5465, 3.4531) (-4.5554, 3.4784) (-4.564, 3.5039) (-4.5725, 3.5295) (-4.5808, 3.5553) (-4.5889, 3.5812) (-4.5968, 3.6072) (-4.6045, 3.6334) (-4.612, 3.6597) (-4.6194, 3.6861) (-4.6265, 3.7127) (-4.6335, 3.7394) (-4.6403, 3.7662) (-4.6468, 3.7932) (-4.6532, 3.8203) (-4.6595, 3.8475) (-4.6655, 3.8749) (-4.6713, 3.9023) (-4.677, 3.9299) (-4.6824, 3.9576) (-4.6877, 3.9854) (-4.6927, 4.0133) (-4.6976, 4.0414) (-4.7023, 4.0695) (-4.7068, 4.0978) (-4.7112, 4.1261) (-4.7153, 4.1546) (-4.7192, 4.1832) (-4.7222, 4.2061) (-4.7244, 4.2234) (-4.7258, 4.2349) (-4.7265, 4.2406) knots 0 0 0 0 0 0 0.01428571 0.02857143 0.04285714 0.05714286 0.07142857 0.08571429 0.1 0.11428571 0.12857143 0.14285714 0.15714286 0.17142857 0.18571429 0.2 0.21428571 0.22857143 0.24285714 0.25714286 0.27142857 0.28571429 0.3 0.31428571 0.32857143 0.34285714 0.35714286 0.37142857 0.38571429 0.4 0.41428571 0.42857143 0.44285714 0.45714286 0.47142857 0.48571429 0.5 0.51428571 0.52857143 0.54285714 0.55714286 0.57142857 0.58571429 0.6 0.61428571 0.62857143 0.64285714 0.65714286 0.67142857 0.68571429 0.7 0.71428571 0.72857143 0.74285714 0.75714286 0.77142857 0.78571429 0.8 0.81428571 0.82857143 0.84285714 0.85714286 0.87142857 0.88571429 0.9 0.91428571 0.92857143 0.94285714 0.95714286 0.97142857 0.98571429 1 1 1 1 1 1
  line L11 (-4.0082, 2.5926) -> (-3.1497, 2.0354)
  arc A23 (-3.0658, 1.6992) -> (-3.1497, 2.0354) centre (-3.288, 1.8223) ccw
  arc A24 (-3.0658, 1.6992) -> (-3.3694, 0.9664) centre (0, 0) ccw
  arc A25 (-3.6664, 0.7879) -> (-3.3694, 0.9664) centre (-3.6135, 1.0364) ccw
  line L12 (-3.6664, 0.7879) -> (-4.6675, 1.001)
  spline S12 degree 5 poles (-4.6675, 1.001) (-4.6721, 1.0019) (-4.6813, 1.0037) (-4.6952, 1.0059) (-4.7138, 1.0078) (-4.7373, 1.0088) (-4.7609, 1.0089) (-4.7846, 1.0084) (-4.8084, 1.0076) (-4.8323, 1.0065) (-4.8562, 1.0051) (-4.8801, 1.0035) (-4.9041, 1.0014) (-4.9282, 0.9988) (-4.9523, 0.9957) (-4.9764, 0.9922) (-5.0006, 0.9883) (-5.0248, 0.9841) (-5.049, 0.9795) (-5.0733, 0.9747) (-5.0975, 0.9696) (-5.1218, 0.9642) (-5.1461, 0.9584) (-5.1705, 0.9524) (-5.1948, 0.946) (-5.2191, 0.9393) (-5.2435, 0.9324) (-5.2679, 0.9251) (-5.2922, 0.9176) (-5.3166, 0.9098) (-5.3409, 0.9017) (-5.3653, 0.8934) (-5.3896, 0.8848) (-5.414, 0.8759) (-5.4383, 0.8668) (-5.4626, 0.8574) (-5.4869, 0.8477) (-5.5112, 0.8378) (-5.5355, 0.8277) (-5.5598, 0.8173) (-5.584, 0.8066) (-5.6082, 0.7957) (-5.6324, 0.7845) (-5.6566, 0.7731) (-5.6808, 0.7615) (-5.7049, 0.7496) (-5.729, 0.7375) (-5.7531, 0.7252) (-5.7771, 0.7126) (-5.8011, 0.6997) (-5.825, 0.6867) (-5.849, 0.6734) (-5.8729, 0.6599) (-5.8967, 0.6462) (-5.9205, 0.6322) (-5.9443, 0.618) (-5.968, 0.6036) (-5.9917, 0.589) (-6.0153, 0.5741) (-6.0389, 0.559) (-6.0625, 0.5438) (-6.086, 0.5282) (-6.1094, 0.5125) (-6.1328, 0.4966) (-6.1561, 0.4804) (-6.1794, 0.464) (-6.2026, 0.4475) (-6.2258, 0.4307) (-6.2489, 0.4137) (-6.2719, 0.3965) (-6.2949, 0.379) (-6.3133, 0.3649) (-6.327, 0.3543) (-6.3361, 0.3471) (-6.3407, 0.3435) knots 0 0 0 0 0 0 0.01428571 0.02857143 0.04285714 0.05714286 0.07142857 0.08571429 0.1 0.11428571 0.12857143 0.14285714 0.15714286 0.17142857 0.18571429 0.2 0.21428571 0.22857143 0.24285714 0.25714286 0.27142857 0.28571429 0.3 0.31428571 0.32857143 0.34285714 0.35714286 0.37142857 0.38571429 0.4 0.41428571 0.42857143 0.44285714 0.45714286 0.47142857 0.48571429 0.5 0.51428571 0.52857143 0.54285714 0.55714286 0.57142857 0.58571429 0.6 0.61428571 0.62857143 0.64285714 0.65714286 0.67142857 0.68571429 0.7 0.71428571 0.72857143 0.74285714 0.75714286 0.77142857 0.78571429 0.8 0.81428571 0.82857143 0.84285714 0.85714286 0.87142857 0.88571429 0.9 0.91428571 0.92857143 0.94285714 0.95714286 0.97142857 0.98571429 1 1 1 1 1 1
  arc A26 (-6.3407, 0.3435) -> (-6.3407, -0.3435) centre (0, 0) ccw
  spline S13 degree 5 poles (-4.6675, -1.001) (-4.6721, -1.0019) (-4.6813, -1.0037) (-4.6952, -1.0059) (-4.7138, -1.0078) (-4.7373, -1.0088) (-4.7609, -1.0089) (-4.7846, -1.0084) (-4.8084, -1.0076) (-4.8323, -1.0065) (-4.8562, -1.0051) (-4.8801, -1.0035) (-4.9041, -1.0014) (-4.9282, -0.9988) (-4.9523, -0.9957) (-4.9764, -0.9922) (-5.0006, -0.9883) (-5.0248, -0.9841) (-5.049, -0.9795) (-5.0733, -0.9747) (-5.0975, -0.9696) (-5.1218, -0.9642) (-5.1461, -0.9584) (-5.1705, -0.9524) (-5.1948, -0.946) (-5.2191, -0.9393) (-5.2435, -0.9324) (-5.2679, -0.9251) (-5.2922, -0.9176) (-5.3166, -0.9098) (-5.3409, -0.9017) (-5.3653, -0.8934) (-5.3896, -0.8848) (-5.414, -0.8759) (-5.4383, -0.8668) (-5.4626, -0.8574) (-5.4869, -0.8477) (-5.5112, -0.8378) (-5.5355, -0.8277) (-5.5598, -0.8173) (-5.584, -0.8066) (-5.6082, -0.7957) (-5.6324, -0.7845) (-5.6566, -0.7731) (-5.6808, -0.7615) (-5.7049, -0.7496) (-5.729, -0.7375) (-5.7531, -0.7252) (-5.7771, -0.7126) (-5.8011, -0.6997) (-5.825, -0.6867) (-5.849, -0.6734) (-5.8729, -0.6599) (-5.8967, -0.6462) (-5.9205, -0.6322) (-5.9443, -0.618) (-5.968, -0.6036) (-5.9917, -0.589) (-6.0153, -0.5741) (-6.0389, -0.559) (-6.0625, -0.5438) (-6.086, -0.5282) (-6.1094, -0.5125) (-6.1328, -0.4966) (-6.1561, -0.4804) (-6.1794, -0.464) (-6.2026, -0.4475) (-6.2258, -0.4307) (-6.2489, -0.4137) (-6.2719, -0.3965) (-6.2949, -0.379) (-6.3133, -0.3649) (-6.327, -0.3543) (-6.3361, -0.3471) (-6.3407, -0.3435) knots 0 0 0 0 0 0 0.01428571 0.02857143 0.04285714 0.05714286 0.07142857 0.08571429 0.1 0.11428571 0.12857143 0.14285714 0.15714286 0.17142857 0.18571429 0.2 0.21428571 0.22857143 0.24285714 0.25714286 0.27142857 0.28571429 0.3 0.31428571 0.32857143 0.34285714 0.35714286 0.37142857 0.38571429 0.4 0.41428571 0.42857143 0.44285714 0.45714286 0.47142857 0.48571429 0.5 0.51428571 0.52857143 0.54285714 0.55714286 0.57142857 0.58571429 0.6 0.61428571 0.62857143 0.64285714 0.65714286 0.67142857 0.68571429 0.7 0.71428571 0.72857143 0.74285714 0.75714286 0.77142857 0.78571429 0.8 0.81428571 0.82857143 0.84285714 0.85714286 0.87142857 0.88571429 0.9 0.91428571 0.92857143 0.94285714 0.95714286 0.97142857 0.98571429 1 1 1 1 1 1
  line L13 (-4.6675, -1.001) -> (-3.6664, -0.7879)
  arc A27 (-3.3694, -0.9664) -> (-3.6664, -0.7879) centre (-3.6135, -1.0364) ccw
  arc A28 (-3.3694, -0.9664) -> (-3.0658, -1.6992) centre (0, 0) ccw
  arc A29 (-3.1497, -2.0354) -> (-3.0658, -1.6992) centre (-3.288, -1.8223) ccw
  line L14 (-3.1497, -2.0354) -> (-4.0082, -2.5926)
  spline S14 degree 5 poles (-4.0082, -2.5926) (-4.0122, -2.5952) (-4.0199, -2.6004) (-4.0313, -2.6087) (-4.0458, -2.6205) (-4.0631, -2.6364) (-4.0799, -2.6531) (-4.0963, -2.6702) (-4.1125, -2.6876) (-4.1286, -2.7053) (-4.1446, -2.7231) (-4.1603, -2.7412) (-4.1758, -2.7596) (-4.191, -2.7785) (-4.2059, -2.7977) (-4.2204, -2.8172) (-4.2348, -2.8371) (-4.2489, -2.8572) (-4.2628, -2.8776) (-4.2766, -2.8981) (-4.2901, -2.9189) (-4.3035, -2.9399) (-4.3166, -2.9612) (-4.3295, -2.9826) (-4.3422, -3.0043) (-4.3547, -3.0263) (-4.367, -3.0484) (-4.3791, -3.0708) (-4.391, -3.0933) (-4.4027, -3.1161) (-4.4142, -3.139) (-4.4256, -3.1621) (-4.4367, -3.1854) (-4.4476, -3.2089) (-4.4584, -3.2326) (-4.4689, -3.2564) (-4.4793, -3.2804) (-4.4895, -3.3046) (-4.4994, -3.329) (-4.5092, -3.3535) (-4.5188, -3.3782) (-4.5283, -3.403) (-4.5375, -3.428) (-4.5465, -3.4531) (-4.5554, -3.4784) (-4.564, -3.5039) (-4.5725, -3.5295) (-4.5808, -3.5553) (-4.5889, -3.5812) (-4.5968, -3.6072) (-4.6045, -3.6334) (-4.612, -3.6597) (-4.6194, -3.6861) (-4.6265, -3.7127) (-4.6335, -3.7394) (-4.6403, -3.7662) (-4.6468, -3.7932) (-4.6532, -3.8203) (-4.6595, -3.8475) (-4.6655, -3.8749) (-4.6713, -3.9023) (-4.677, -3.9299) (-4.6824, -3.9576) (-4.6877, -3.9854) (-4.6927, -4.0133) (-4.6976, -4.0414) (-4.7023, -4.0695) (-4.7068, -4.0978) (-4.7112, -4.1261) (-4.7153, -4.1546) (-4.7192, -4.1832) (-4.7222, -4.2061) (-4.7244, -4.2234) (-4.7258, -4.2349) (-4.7265, -4.2406) knots 0 0 0 0 0 0 0.01428571 0.02857143 0.04285714 0.05714286 0.07142857 0.08571429 0.1 0.11428571 0.12857143 0.14285714 0.15714286 0.17142857 0.18571429 0.2 0.21428571 0.22857143 0.24285714 0.25714286 0.27142857 0.28571429 0.3 0.31428571 0.32857143 0.34285714 0.35714286 0.37142857 0.38571429 0.4 0.41428571 0.42857143 0.44285714 0.45714286 0.47142857 0.48571429 0.5 0.51428571 0.52857143 0.54285714 0.55714286 0.57142857 0.58571429 0.6 0.61428571 0.62857143 0.64285714 0.65714286 0.67142857 0.68571429 0.7 0.71428571 0.72857143 0.74285714 0.75714286 0.77142857 0.78571429 0.8 0.81428571 0.82857143 0.84285714 0.85714286 0.87142857 0.88571429 0.9 0.91428571 0.92857143 0.94285714 0.95714286 0.97142857 0.98571429 1 1 1 1 1 1
  arc A30 (-4.7265, -4.2406) -> (-4.2406, -4.7265) centre (0, 0) ccw
  spline S15 degree 5 poles (-2.5926, -4.0082) (-2.5952, -4.0122) (-2.6004, -4.0199) (-2.6087, -4.0313) (-2.6205, -4.0458) (-2.6364, -4.0631) (-2.6531, -4.0799) (-2.6702, -4.0963) (-2.6876, -4.1125) (-2.7053, -4.1286) (-2.7231, -4.1446) (-2.7412, -4.1603) (-2.7596, -4.1758) (-2.7785, -4.191) (-2.7977, -4.2059) (-2.8172, -4.2204) (-2.8371, -4.2348) (-2.8572, -4.2489) (-2.8776, -4.2628) (-2.8981, -4.2766) (-2.9189, -4.2901) (-2.9399, -4.3035) (-2.9612, -4.3166) (-2.9826, -4.3295) (-3.0043, -4.3422) (-3.0263, -4.3547) (-3.0484, -4.367) (-3.0708, -4.3791) (-3.0933, -4.391) (-3.1161, -4.4027) (-3.139, -4.4142) (-3.1621, -4.4256) (-3.1854, -4.4367) (-3.2089, -4.4476) (-3.2326, -4.4584) (-3.2564, -4.4689) (-3.2804, -4.4793) (-3.3046, -4.4895) (-3.329, -4.4994) (-3.3535, -4.5092) (-3.3782, -4.5188) (-3.403, -4.5283) (-3.428, -4.5375) (-3.4531, -4.5465) (-3.4784, -4.5554) (-3.5039, -4.564) (-3.5295, -4.5725) (-3.5553, -4.5808) (-3.5812, -4.5889) (-3.6072, -4.5968) (-3.6334, -4.6045) (-3.6597, -4.612) (-3.6861, -4.6194) (-3.7127, -4.6265) (-3.7394, -4.6335) (-3.7662, -4.6403) (-3.7932, -4.6468) (-3.8203, -4.6532) (-3.8475, -4.6595) (-3.8749, -4.6655) (-3.9023, -4.6713) (-3.9299, -4.677) (-3.9576, -4.6824) (-3.9854, -4.6877) (-4.0133, -4.6927) (-4.0414, -4.6976) (-4.0695, -4.7023) (-4.0978, -4.7068) (-4.1261, -4.7112) (-4.1546, -4.7153) (-4.1832, -4.7192) (-4.2061, -4.7222) (-4.2234, -4.7244) (-4.2349, -4.7258) (-4.2406, -4.7265) knots 0 0 0 0 0 0 0.01428571 0.02857143 0.04285714 0.05714286 0.07142857 0.08571429 0.1 0.11428571 0.12857143 0.14285714 0.15714286 0.17142857 0.18571429 0.2 0.21428571 0.22857143 0.24285714 0.25714286 0.27142857 0.28571429 0.3 0.31428571 0.32857143 0.34285714 0.35714286 0.37142857 0.38571429 0.4 0.41428571 0.42857143 0.44285714 0.45714286 0.47142857 0.48571429 0.5 0.51428571 0.52857143 0.54285714 0.55714286 0.57142857 0.58571429 0.6 0.61428571 0.62857143 0.64285714 0.65714286 0.67142857 0.68571429 0.7 0.71428571 0.72857143 0.74285714 0.75714286 0.77142857 0.78571429 0.8 0.81428571 0.82857143 0.84285714 0.85714286 0.87142857 0.88571429 0.9 0.91428571 0.92857143 0.94285714 0.95714286 0.97142857 0.98571429 1 1 1 1 1 1
  line L15 (-2.5926, -4.0082) -> (-2.0354, -3.1497)
  arc A31 (-1.6992, -3.0658) -> (-2.0354, -3.1497) centre (-1.8223, -3.288) ccw
  arc A32 (-1.6992, -3.0658) -> (-0.9664, -3.3694) centre (0, 0) ccw
  circle A33 centre (0, 0) radius 6.35
  circle A34 centre (0, 0) radius 3.175
  constraint concentric A0 A33
  constraint coincident S4.end A33
extrude "Extrude3" add sketch "Sketch3 (2)" along normal blind 5.08 in component "Spur Gear (8 teeth)"
chamfer "Chamfer1" distance 0.127 distance2 12.7 1 edges at (2.9601, 1.1481, -5.08) measured on face at (2.6575, -4.5647, -5.08) in component "Spur Gear (8 teeth)"
chamfer "Chamfer2" distance 0.508 distance2 0.762 1 edges at (3.0785, -1.1941, -5.08) measured on face at (-1.7101, 2.775, -0.8475) in component "Spur Gear (8 teeth)"
component "Spur Gear (8 teeth)" placed x (1, 0, 0) y (0, 1, 0) z (0, 0, 1) at (0, 0, 0)
